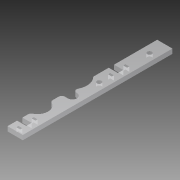
# Autodesk Inventor part: plastic_part_53
Saved by Autodesk Inventor 2013 (Build 170138000, 138)
## iProperties
Shininess: 20.0
Created: 2014-03-15
Part Number: plastic_part_53
Document SubType Name: Modeling
Designer: Noa Izumi
Material: Default
Density: 1 g/cm^3
Density: 0.0
Volumn: 0.0
Area: 0.0
PropertySet Name: Model Information
Control State: 0
Master: False
Checked Out: False
Author: Noa Izumi
Autodesk Inventor part; units mm, degrees
ref_plane "YZ Plane" through (0, 0, 0) normal (1, 0, 0) x (0, 1, 0)
ref_plane "XZ Plane" through (0, 0, 0) normal (0, 1, 0) x (-1, 0, 0)
ref_plane "XY Plane" through (0, 0, 0) normal (0, 0, 1) x (1, 0, 0)
sketch "Sketch1" plane through (0, 0, 0) normal (0, 0, 1) x (1, 0, 0)
  line L0 (0, 0) -> (10, 0)
  line L1 (10, 0) -> (10, 98)
  line L2 (10, 98) -> (0, 98)
  line L3 (0, 98) -> (0, 0)
  line L4 (0, 9.7325) -> (6, 9.7325)
  line L5 (6, 9.7325) -> (6, 6.2675)
  line L6 (6, 6.2675) -> (0, 6.2675)
  line L7 (0, 6.2675) -> (0, 9.7325)
  line L8 (0, 69.7325) -> (6, 69.7325)
  line L9 (6, 69.7325) -> (6, 66.2675)
  line L10 (6, 66.2675) -> (0, 66.2675)
  line L11 (0, 66.2675) -> (0, 69.7325)
  dimension "d0" = 10
  dimension "d1" = 98
  dimension "d10" = 6.2675
  dimension "d11" = 3.465
  dimension "d12" = 6
  dimension "d13" = 3.465
  dimension "d14" = 28.2675
  dimension "d15" = 6
  constraints: 24 end point, 6 parallel, 3 horizontal, 3 perpendicular, 2 point on line
  measures "d0" distance of L0.start L0.end
  measures "d1" distance of L2.end L0.start
  measures "d10" distance between parallel lines of L0 L6
  measures "d11" distance of L4.end L5.end
  measures "d12" distance of L5.end L6.end
  measures "d13" distance of L8.end L9.end
  measures "d14" distance between parallel lines of L8 L2
  measures "d15" distance of L9.end L10.end
extrude "Extrusion1" add sketch "Sketch1" along normal blind 3 contours L3 L6 L5 L4 L10 L9 L8 L2 L1 L0
sketch "Sketch2" plane through (0, 0, 3) normal (0, 0, 1) x (1, 0, 0)
  line L0 (10, 0) -> (0, 0) projected
  line L1 (10, 98) -> (10, 0) projected
  line L2 (0, 98) -> (10, 98) projected
  line L3 (6, 69.7325) -> (6, 66.2675) projected
  line L4 (6, 3.7) -> (3.5, 3.7)
  line L5 (3.5, 3.7) -> (3.5, 2.3)
  line L6 (3.5, 2.3) -> (6, 2.3)
  line L7 (6, 2.3) -> (6, 3.7)
  line L8 (6, 12.3) -> (3.5, 12.3)
  line L9 (3.5, 12.3) -> (3.5, 13.7)
  line L10 (3.5, 13.7) -> (6, 13.7)
  line L11 (6, 13.7) -> (6, 12.3)
  line L12 (6, 63.7) -> (3.5, 63.7)
  line L13 (3.5, 63.7) -> (3.5, 62.3)
  line L14 (3.5, 62.3) -> (6, 62.3)
  line L15 (6, 62.3) -> (6, 63.7)
  line L16 (6, 72.3) -> (3.5, 72.3)
  line L17 (3.5, 72.3) -> (3.5, 73.7)
  line L18 (3.5, 73.7) -> (6, 73.7)
  line L19 (6, 73.7) -> (6, 72.3)
  dimension "d16" = 1.4
  dimension "d17" = 2.5
  dimension "d18" = 2.3
  dimension "d19" = 1.4
  dimension "d20" = 8.6
  dimension "d21" = 2.5
  dimension "d22" = 4
  dimension "d23" = 1.4
  dimension "d24" = 1.4
  dimension "d25" = 2.5
  dimension "d26" = 24.3
  dimension "d27" = 8.6
  constraints: 32 end point, 8 parallel, 4 horizontal, 4 perpendicular, 1 point on line
  measures "d16" distance of L6.end L4.start
  measures "d17" distance of L5.end L6.end
  measures "d18" distance between parallel lines of L0 L6
  measures "d19" distance of L10.end L8.start
  measures "d20" distance between parallel lines of L4 L8
  measures "d21" distance of L13.end L14.end
  measures "d22" distance between parallel lines of L1 L15
  measures "d23" distance of L14.end L12.start
  measures "d24" distance of L18.end L16.start
  measures "d25" distance of L17.end L18.end
  measures "d26" distance between parallel lines of L2 L18
  measures "d27" distance between parallel lines of L12 L16
extrude "Extrusion2" cut sketch "Sketch2" against normal through all
sketch "草圖7" plane through (0, 0, 3) normal (0, 0, 1) x (1, 0, 0)
  line L0 (0, 98) -> (10, 98) projected
  point P0 (5, 88)
  point P1 (5, 55)
  dimension "d67" = 10
  dimension "d68" = 43
  measures "d67" distance from line of L0 point (5, 88)
  measures "d68" distance from line of L0 point (5, 55)
hole "孔4" at (5, 88, 3) at (5, 55, 3) direction (0, 0, -1) diameter 3 end through all
sketch "草圖8" plane through (0, 0, 3) normal (0, 0, 1) x (1, 0, 0)
  line L0 (0, 9.7325) -> (0, 66.2675) projected
  line L1 (10, 0) -> (0, 0) projected
  line L2 (10, 98) -> (10, 0) projected
  line L3 (0, 98) -> (10, 98) projected
  circle A0 centre (-7, 49) radius 10
  circle A1 centre (-2, 21.5) radius 7
  circle A2 centre (4, 38.5) radius 3
  line L4 (4, 41.5) -> (0, 41.5)
  line L5 (0, 41.5) -> (0, 35.5)
  line L6 (0, 35.5) -> (4, 35.5)
  line L7 (4, 35.5) -> (4, 41.5)
  dimension "d84" = 6
  dimension "d76" = 49
  dimension "d77" = 7
  dimension "d78" = 20
  dimension "d79" = 12
  dimension "d80" = 21.5
  dimension "d81" = 14
  dimension "d82" = 38.5
  dimension "d83" = 6
  constraints: 8 end point, 2 centre point, 2 parallel, 1 horizontal, 1 perpendicular, 1 point on line, 1 vertical alignment, 2 other
  measures "d76" distance from line of L3 A0.centre
  measures "d77" distance from line of L0 A0.centre
  measures "d78" diameter of A0
  measures "d79" distance from line of L2 A1.centre
  measures "d80" distance from line of L1 A1.centre
  measures "d81" diameter of A1
  measures "d82" distance from line of L1 point (4, 38.5)
  measures "d83" distance from line of L2 point (4, 38.5)
extrude "擠出4" cut sketch "草圖8" against normal through all
fillet "圓角4" radius 2 5 edges at (0, 14.7918, 1.5) (0, 28.2082, 1.5) (0, 35.5, 1.5) (0, 41.5, 1.5) (0, 41.8586, 1.5)
